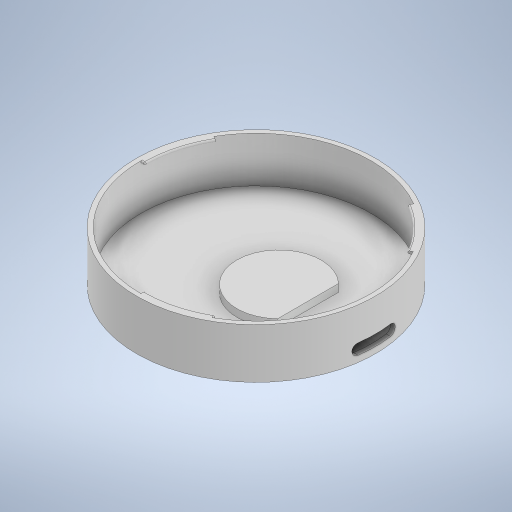
# Autodesk Inventor part: bottom_basket_2
Saved by Autodesk Inventor 2023 (Build 270158000, 158)
## iProperties
Created: 2025-12-29
Part Number: bottom_basket_2
Material: Generic
Document SubType Name: Modeling
Designer: Justin Pascual
Density: 1 g/cm^3
Appearance: Default
Author: Justin Pascual
Autodesk Inventor part; units mm, degrees
ref_plane "YZ Plane" through (0, 0, 0) normal (1, 0, 0) x (0, 1, 0)
ref_plane "XZ Plane" through (0, 0, 0) normal (0, 1, 0) x (-1, 0, 0)
ref_plane "XY Plane" through (0, 0, 0) normal (0, 0, 1) x (1, 0, 0)
sketch "Sketch1" plane through (0, 0, 0) normal (0, 1, 0) x (-1, 0, 0)
  circle A0 centre (0, 0) radius 69.85
  dimension "d0" = 139.7
  constraints: 1 centre point, 1 coincident
  measures "d0" diameter of A0
extrude "Extrusion1" add sketch "Sketch1" along normal blind 29.21
sketch "Sketch3" plane through (0, 29.21, 0) normal (0, 1, 0) x (1, 0, 0)
  circle A0 centre (0, 0) radius 67.31
  dimension "d5" = 134.62
  constraints: 1 centre point, 1 coincident
  measures "d5" diameter of A0
extrude "Extrusion2" cut sketch "Sketch3" against normal blind 26.67
sketch "Sketch6" plane through (0, 0, 0) normal (1, 0, 0) x (0, 1, 0)
  line L0 (29.21, 67.31) -> (2.54, 67.31) projected
  line L1 (29.21, 67.31) -> (27.686, 67.31)
  line L2 (27.686, 67.31) -> (27.686, 65.024)
  line L3 (27.686, 65.024) -> (29.21, 65.024)
  line L4 (29.21, 65.024) -> (29.21, 67.31)
  line L5 (-5.842, 0) -> (35.052, 0) projected
  line L6 (29.21, -69.85) -> (29.21, 69.85) projected
  point P0 (0, 0)
  dimension "d21" = 1.524
  dimension "d22" = 2.286
  dimension "d36" = 0
  constraints: 8 end point, 2 parallel, 1 horizontal, 1 perpendicular, 1 point on line
  measures "d21" distance of L3.end L2.end
  measures "d22" distance of L2.end L1.end
  measures "d36" distance between parallel lines of L6 L4
revolve "Revolution1" add sketch "Sketch6" angle 30 about axis through (0, -10, 0) along (0, 1, 0)
fillet "Fillet2" radius 0.762 2 edges at (16.8294, 27.686, 62.8084) (16.8294, 29.21, 62.8084)
fillet "Fillet3" radius 0.762 3 edges at (32.6235, 27.909, 56.5056) (33.2739, 29.21, 57.632) (33.2739, 27.686, 57.632)
pattern_circular "Circular Pattern1" count 3 over 360 about axis through (0, 0, 0) along (0, 1, 0) of "Revolution1", "Fillet2", "Fillet3"
sketch "Sketch9" plane through (0, 0, 0) normal (1, 0, 0) x (0, 1, 0)
  circle A0 centre (6.8717, 0) radius 3.175 construction
  line L0 (6.8717, 0) -> (6.8717, -12.7) construction
  line L1 (6.8717, 0) -> (6.8717, 12.7) construction
  line L2 (6.8717, -12.7) -> (6.8717, -12.7)
  line L3 (3.6967, -9.525) -> (3.6967, 9.525)
  line L4 (6.8717, 12.7) -> (6.8717, 12.7)
  line L5 (10.0467, 9.525) -> (10.0467, -9.525)
  arc A1 (6.8717, -12.7) -> (10.0467, -9.525) centre (6.8717, -9.525) ccw
  arc A2 (3.6967, -9.525) -> (6.8717, -12.7) centre (6.8717, -9.525) ccw
  arc A3 (6.8717, 12.7) -> (3.6967, 9.525) centre (6.8717, 9.525) ccw
  arc A4 (10.0467, 9.525) -> (6.8717, 12.7) centre (6.8717, 9.525) ccw
  point P0 (0, 0)
  dimension "d37" = 6.35
  dimension "d48" = 12.7
  dimension "d49" = 12.7
  dimension "d50" = 3.175
  constraints: 12 end point, 8 point on circle, 8 tangent, 5 centre point, 3 equal radius, 2 parallel, 1 horizontal, 1 perpendicular, 1 point on line, 1 vertical
  measures "d37" diameter of A0
  measures "d48" distance of L0.start L0.end
  measures "d49" distance of L0.start L1.end
  measures "d50" radius of A1
extrude "Extrusion9" cut sketch "Sketch9" along normal through all
sketch "Sketch20" plane through (0, 2.54, 0) normal (0, 1, 0) x (1, 0, 0)
  circle A0 centre (0, 0) radius 3.4925
  circle A1 centre (13.4366, 0) radius 24.638
  line L0 (38.0746, 0) -> (30.4546, 0) construction
  line L1 (30.4546, 0) -> (30.4546, -17.8162)
  line L2 (30.4546, 0) -> (30.4546, 17.8162)
  dimension "d70" = 6.985
  dimension "d71" = 49.276
  dimension "d72" = 13.4366
  dimension "d73" = 7.62
  constraints: 6 end point, 3 point on circle, 2 centre point, 2 vertical, 1 coincident, 1 horizontal
  measures "d70" diameter of A0
  measures "d71" diameter of A1
  measures "d72" distance of point (0, 0) A1.centre
  measures "d73" distance of L0.start L0.end
extrude "Extrusion13" add sketch "Sketch20" along normal blind 4.445 contours A0 | L2 L1 A1 picked at (19.7197, -7.6808)
body "Solid1"
